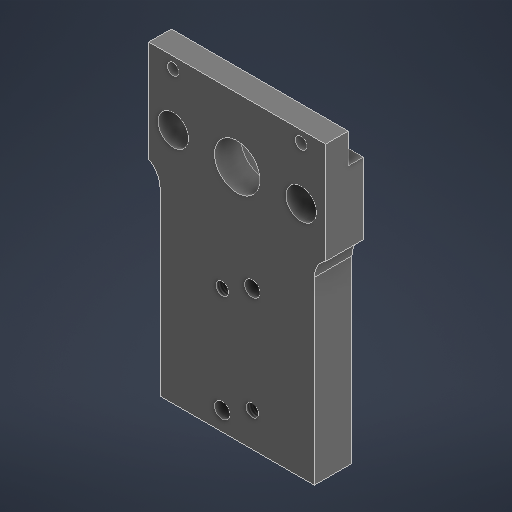
# Autodesk Inventor part: Lap2
Saved by Autodesk Inventor 2025 (Build 290162010, 162A)
## iProperties
Created: 2025-01-17
Part Number: Lap2
Material: Steel, Carbon
Document SubType Name: Modeling
Designer: Tanár
Density: 7.85 g/cm^3
Appearance: Gray
Author: Tanár
Autodesk Inventor part; units mm, degrees
ref_plane "YZ Plane" through (0, 0, 0) normal (1, 0, 0) x (0, 1, 0)
ref_plane "XZ Plane" through (0, 0, 0) normal (0, 1, 0) x (-1, 0, 0)
ref_plane "XY Plane" through (0, 0, 0) normal (0, 0, 1) x (1, 0, 0)
sketch "Sketch1" plane through (0, 0, 0) normal (0, 0, 1) x (1, 0, 0)
  line L0 (0, 40) -> (0, -40)
  line L1 (0, 40) -> (23.5, 40)
  line L2 (23.5, 40) -> (23.5, 13)
  arc A0 (23.5, 13) -> (20.5, 7.8038) centre (26.5, 7.8038) ccw
  line L3 (20.5, 7.8038) -> (20.5, -40)
  line L4 (20.5, -40) -> (0, -40)
  line L5 (0, 40) -> (-23.5, 40)
  line L6 (-23.5, 40) -> (-23.5, 13)
  arc A1 (-20.5, 7.8038) -> (-23.5, 13) centre (-26.5, 7.8038) ccw
  line L7 (-20.5, 7.8038) -> (-20.5, -40)
  line L8 (-20.5, -40) -> (0, -40)
  point P0 (0, 0)
  point P1 (0, 0)
  point P2 (10.25, -40)
  dimension "d0" = 47
  dimension "d1" = 80
  dimension "d2" = 27
  dimension "d3" = 41
  dimension "d4" = 6
  constraints: 18 end point, 5 symmetric about line, 4 point on circle, 2 centre point, 2 midpoint, 2 perpendicular, 2 vertical, 1 coincident, 1 horizontal, 1 tangent, 1 other
  measures "d0" diameter of L2 L0
  measures "d1" distance from line of point (10.25, -40) L1
  measures "d2" distance of L1.end L2.end
  measures "d3" diameter of L3 L0
  measures "d4" radius of A0
extrude "Extrusion1" add sketch "Sketch1" along normal mid plane 10
sketch "Sketch2" plane through (23.5, 13, 5) normal (1, 0, 0) x (0, 0, -1)
  line L0 (10, 27) -> (0, 27) projected
  line L1 (6, 27) -> (6, 19)
  line L2 (6, 19) -> (10, 19)
  line L3 (10, 27) -> (10, 0) projected
  point P0 (5, -13)
  dimension "d7" = 8
  dimension "d8" = 4
  constraints: 4 end point, 2 point on line, 1 perpendicular, 1 vertical
  measures "d7" distance of L1.start L1.end
  measures "d8" distance of L1.end L2.end
extrude "Extrusion2" cut sketch "Sketch2" against normal through all
sketch "Sketch3" plane through (0, 0, -5) normal (0, 0, -1) x (-1, 0, 0)
  line L0 (-23.5, 40) -> (23.5, 40) projected
  line L1 (0, 40) -> (0, -40)
  line L2 (-20.5, -40) -> (20.5, -40) projected
  line L3 (-20.5, 7.8038) -> (-20.5, -40) projected
  point P0 (0, 0)
  point P1 (-17, 23)
  point P2 (0, 23)
  point P3 (17, 23)
  point P4 (-4, -3)
  point P5 (4, -7)
  point P6 (-4, -31)
  point P7 (4, -35)
  dimension "d11" = 17
  dimension "d12" = 34
  dimension "d13" = 5
  dimension "d14" = 32
  dimension "d15" = 4
  dimension "d16" = 24
  dimension "d17" = 16.5
  dimension "d18" = 24.5
  constraints: 3 vertical alignment, 2 end point, 2 horizontal alignment, 2 midpoint, 1 symmetric about line
  measures "d11" distance from line of L0 point (17, 23)
  measures "d12" distance of point (17, 23) point (-17, 23)
  measures "d13" distance from line of point (4, -35) L2
  measures "d14" vertical distance of point (-4, -3) point (4, -35)
  measures "d15" vertical distance of point (4, -7) point (-4, -3)
  measures "d16" vertical distance of point (-4, -31) point (4, -7)
  measures "d17" distance from line of point (-4, -31) L3
  measures "d18" distance from line of L3 point (4, -35)
hole "Hole1" at (-4, -35, -5) at (4, -3, -5) direction (0, 0, 1) diameter 4 end through all
hole "Hole2" at (4, -31, -5) at (-4, -7, -5) direction (0, 0, 1) diameter 3.242 end through all thread size "M4x0.7" class "6H" standard "ISO Metric profile"
hole "Hole3" at (17, 23, -5) at (-17, 23, -5) direction (0, 0, 1) diameter 8 end through all
hole "Hole4" at (0, 23, -5) direction (0, 0, 1) diameter 12 end through all counterbore diameter 16 counterbore depth 3
sketch "Sketch5" plane through (23.5, 32, -1) normal (0, 0, -1) x (-1, 0, 0)
  line L0 (0, 8) -> (47, 8) projected
  line L1 (23.5, 8) -> (23.5, 5)
  line L2 (23.5, 5) -> (40.5, 5)
  line L3 (40.5, 5) -> (6.5, 5)
  circle A0 centre (6.5, 5) radius 1.5
  circle A1 centre (40.5, 5) radius 1.5
  point P0 (23.5, -32)
  dimension "d58" = 3
  dimension "d59" = 17
  dimension "d60" = 34
  dimension "d61" = 3
  dimension "d62" = 3
  constraints: 6 end point, 2 centre point, 2 coincident, 1 midpoint, 1 perpendicular, 1 point on line, 1 vertical
  measures "d58" distance of L1.start L1.end
  measures "d59" distance of L1.end L2.end
  measures "d60" distance of L2.end L3.end
  measures "d61" diameter of A0
  measures "d62" diameter of A1
extrude "Extrusion4" cut sketch "Sketch5" against normal blind 10
body "Solid1"
